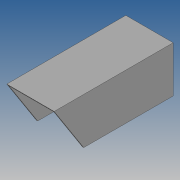
# Autodesk Inventor part: P034_Casquette
Saved by Autodesk Inventor 2021.3 (Build 253353000, 353)
## iProperties
Created: 2021-11-26
Part Number: P034_Casquette
Material: Générique
Document SubType Name: Modeling
Designer: gabri
Density: 1 g/cm^3
Appearance: Par défaut
Author: gabri
Autodesk Inventor part; units mm, degrees
ref_plane "YZ Plane" through (0, 0, 0) normal (1, 0, 0) x (0, 1, 0)
ref_plane "XZ Plane" through (0, 0, 0) normal (0, 1, 0) x (-1, 0, 0)
ref_plane "XY Plane" through (0, 0, 0) normal (0, 0, 1) x (1, 0, 0)
sketch "Sketch2" plane through (0, 0, 0) normal (0, 0, 1) x (1, 0, 0)
  line L0 (53, 53) -> (-53, 53)
  line L1 (-53, 53) -> (-53, -53)
  line L2 (-53, -53) -> (53, -53)
  line L3 (53, -53) -> (53, 53)
  line L4 (53, 53) -> (-53, -53) construction
  line L5 (-53, 53) -> (53, -53) construction
  point P0 (0, 0)
  dimension "d0" = 106
  dimension "d1" = 106
  constraints: 12 end point, 2 midpoint, 2 parallel, 1 horizontal, 1 perpendicular
  measures "d0" distance of L2.end L1.end
  measures "d1" distance between parallel lines of L0 L2
extrude "Extrusion1" add sketch "Sketch2" along normal blind 103
sketch "Sketch3" plane through (-53, -53, 0) normal (0, -1, 0) x (1, 0, 0)
  line L0 (0, 0) -> (106, 0) construction
  line L1 (106, 0) -> (106, 103) construction
  line L2 (0, 103) -> (106, 103) construction
  line L3 (0, 0) -> (0, 103) construction
  line L4 (103, 0) -> (3, 0)
  line L5 (3, 0) -> (3, 100)
  line L6 (3, 100) -> (103, 100)
  line L7 (103, 100) -> (103, 0)
  line L8 (103, 0) -> (3, 100) construction
  line L9 (3, 0) -> (103, 100) construction
  line L10 (53, 127.2) -> (53, -21.2) construction
  point P0 (53, 0)
  point P1 (53, 50)
  point P2 (53, 50)
  point P3 (53, 0)
  dimension "d4" = 3
  dimension "d5" = 3
  constraints: 12 end point, 5 midpoint, 2 parallel, 1 horizontal, 1 perpendicular, 1 point on line
  measures "d4" distance between parallel lines of L2 L6
  measures "d5" distance between parallel lines of L1 L7
extrude "Extrusion2" cut sketch "Sketch3" against normal up to surface (106 mm away)
sketch "Sketch4" plane through (53, -53, 0) normal (1, 0, 0) x (0, 0, -1)
  line L0 (0, 0) -> (0, 106) construction
  line L1 (0, 106) -> (-103, 106) construction
  line L2 (-103, 0) -> (-103, 106) construction
  line L3 (0, 0) -> (-103, 0) construction
  line L4 (0, 0) -> (-103, 0)
  line L5 (-103, 0) -> (0, 66)
  line L6 (0, 0) -> (0, 66)
  point P0 (0, 53)
  dimension "d14" = 40
  constraints: 6 end point, 2 collinear, 1 point on line
  measures "d14" distance from line of L1 L5.end
extrude "Extrusion3" cut sketch "Sketch4" against normal up to surface (106 mm away)
sketch "Sketch5" plane through (-53, 53, 103) normal (0, 1, 0) x (1, 0, 0)
  line L0 (3, 3) -> (3, 103) construction
  line L1 (0, 103) -> (0, 0) construction
  line L2 (106, 0) -> (0, 0) construction
  line L3 (106, 103) -> (106, 0) construction
  line L4 (103, 103) -> (103, 3) construction
  line L5 (103, 3) -> (3, 3) construction
  line L6 (103, 103) -> (106, 103)
  line L7 (106, 103) -> (106, 0)
  line L8 (0, 0) -> (0, 103)
  line L9 (3, 103) -> (0, 103)
  line L10 (3, 103) -> (3, 3)
  line L11 (3, 3) -> (103, 3)
  line L12 (103, 3) -> (103, 103)
  line L13 (106, 0) -> (0, 0)
  line L14 (127.2, 103) -> (-21.2, 103) construction
  line L15 (3, 103) -> (0, 103) projected
  line L16 (106, 103) -> (103, 103) projected
  point P0 (53, 103)
  point P1 (1.5, 103)
  constraints: 16 end point, 5 collinear, 3 perpendicular, 1 midpoint, 1 point on line
extrude "Extrusion4" add sketch "Sketch5" along normal blind 160
body "Solid1"
